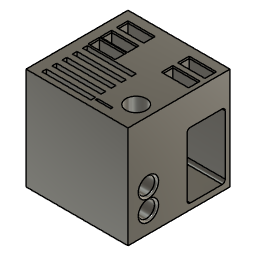
porte_carte_usb v3 (Autodesk Fusion 360 design; units mm, degrees)
Autodesk Fusion 360 part; units mm, degrees
note: some values were not read from the file. Set by a fixed rule: which sketch regions a step uses.
sketch "Esquisse1" plane through (0, 0, 0) normal (0, 0, 1) x (1, 0, 0)
  line L0 (0, 0) -> (50, 0)
  line L1 (50, 0) -> (50, 50)
  line L2 (50, 50) -> (0, 50)
  line L3 (0, 50) -> (0, 0)
  dimension "d1" = 50
  dimension "d2" = 50
  constraint horizontal L0
  constraint vertical L1
  constraint horizontal L2
  constraint vertical L3
  constraint coincident L0.start L3.end
  measures "d1" distance of L0.start L0.end
  measures "d2" distance of L0.start L2.end
extrude "Extrusion1" add sketch "Esquisse1" along normal blind 50
sketch "Esquisse2" plane through (0, 0, 50) normal (0, 0, 1) x (-1, 0, 0)
  line L0 (0, -50) -> (0, 0)
  line L1 (0, 0) -> (-50, 0)
  line L2 (-50, 0) -> (-50, -50)
  line L3 (-50, -50) -> (0, -50)
  line L4 (-5, -45) -> (-17.3, -45)
  line L5 (-17.3, -45) -> (-17.3, -40.4)
  line L6 (-17.3, -40.4) -> (-5, -40.4)
  line L7 (-5, -40.4) -> (-5, -45)
  line L8 (-35, -45) -> (-47.3, -45)
  line L9 (-47.3, -45) -> (-47.3, -40.4)
  line L10 (-47.3, -40.4) -> (-35, -40.4)
  line L11 (-35, -40.4) -> (-35, -45)
  line L12 (-5, -37) -> (-17.3, -37)
  line L13 (-17.3, -37) -> (-17.3, -32.4)
  line L14 (-17.3, -32.4) -> (-5, -32.4)
  line L15 (-5, -32.4) -> (-5, -37)
  line L16 (-35, -37) -> (-47.3, -37)
  line L17 (-47.3, -37) -> (-47.3, -32.4)
  line L18 (-47.3, -32.4) -> (-35, -32.4)
  line L19 (-35, -32.4) -> (-35, -37)
  line L20 (-5, -25) -> (-29, -25)
  line L21 (-29, -25) -> (-29, -22.8)
  line L22 (-29, -22.8) -> (-5, -22.8)
  line L23 (-5, -22.8) -> (-5, -25)
  line L24 (-5, -20) -> (-29, -20)
  line L25 (-29, -20) -> (-29, -17.8)
  line L26 (-29, -17.8) -> (-5, -17.8)
  line L27 (-5, -17.8) -> (-5, -20)
  line L28 (-5, -15) -> (-29, -15)
  line L29 (-29, -15) -> (-29, -12.8)
  line L30 (-29, -12.8) -> (-5, -12.8)
  line L31 (-5, -12.8) -> (-5, -15)
  line L32 (-5, -10) -> (-29, -10)
  line L33 (-29, -10) -> (-29, -7.8)
  line L34 (-29, -7.8) -> (-5, -7.8)
  line L35 (-5, -7.8) -> (-5, -10)
  line L36 (-5, -5) -> (-29, -5)
  line L37 (-29, -5) -> (-29, -2.8)
  line L38 (-29, -2.8) -> (-5, -2.8)
  line L39 (-5, -2.8) -> (-5, -5)
  line L40 (-30, -30) -> (-37, -30)
  line L41 (-37, -30) -> (-37, -29)
  line L42 (-37, -29) -> (-30, -29)
  line L43 (-30, -29) -> (-30, -30)
  line L44 (-41, -30) -> (-47, -30)
  line L45 (-47, -30) -> (-47, -29)
  line L46 (-47, -29) -> (-41, -29)
  line L47 (-41, -29) -> (-41, -30)
  line L48 (-30, -25) -> (-37, -25)
  line L49 (-37, -25) -> (-37, -24)
  line L50 (-37, -24) -> (-30, -24)
  line L51 (-30, -24) -> (-30, -25)
  line L52 (-41, -25) -> (-47, -25)
  line L53 (-47, -25) -> (-47, -24)
  line L54 (-47, -24) -> (-41, -24)
  line L55 (-41, -24) -> (-41, -25)
  line L56 (-30, -20) -> (-37, -20)
  line L57 (-37, -20) -> (-37, -19)
  line L58 (-37, -19) -> (-30, -19)
  line L59 (-30, -19) -> (-30, -20)
  line L60 (-41, -20) -> (-47, -20)
  line L61 (-47, -20) -> (-47, -19)
  line L62 (-47, -19) -> (-41, -19)
  line L63 (-41, -19) -> (-41, -20)
  line L64 (-30, -5) -> (-37.6, -5)
  line L65 (-37.6, -5) -> (-37.6, -4)
  line L66 (-37.6, -4) -> (-30, -4)
  line L67 (-30, -4) -> (-30, -5)
  circle A0 centre (-42, -12) radius 5
  line L68 (-5, -31) -> (-17.3, -31)
  line L69 (-17.3, -31) -> (-17.3, -26.4)
  line L70 (-17.3, -26.4) -> (-5, -26.4)
  line L71 (-5, -26.4) -> (-5, -31)
  circle A1 centre (-33.8, -4.5) radius 0.5
  dimension "d15" = 4.6
  dimension "d16" = 12.3
  dimension "d17" = 12.3
  dimension "d18" = 4.6
  dimension "d19" = 12.3
  dimension "d20" = 4.6
  dimension "d21" = 12.3
  dimension "d22" = 4.6
  dimension "d23" = 24
  dimension "d24" = 2.2
  dimension "d25" = 24
  dimension "d26" = 2.2
  dimension "d27" = 24
  dimension "d28" = 2.2
  dimension "d29" = 24
  dimension "d30" = 2.2
  dimension "d31" = 24
  dimension "d32" = 2.2
  dimension "d33" = 7.6
  dimension "d34" = 1
  dimension "d35" = 12.3
  dimension "d36" = 4.6
  constraint horizontal L4
  constraint vertical L5
  constraint horizontal L6
  constraint vertical L7
  constraint horizontal L8
  constraint vertical L9
  constraint horizontal L10
  constraint vertical L11
  constraint horizontal L12
  constraint vertical L13
  constraint horizontal L14
  constraint vertical L15
  constraint horizontal L16
  constraint vertical L17
  constraint horizontal L18
  constraint vertical L19
  constraint horizontal L20
  constraint vertical L21
  constraint horizontal L22
  constraint vertical L23
  constraint horizontal L24
  constraint vertical L25
  constraint horizontal L26
  constraint vertical L27
  constraint horizontal L28
  constraint vertical L29
  constraint horizontal L30
  constraint vertical L31
  constraint horizontal L32
  constraint vertical L33
  constraint horizontal L34
  constraint vertical L35
  constraint horizontal L36
  constraint vertical L37
  constraint horizontal L38
  constraint vertical L39
  constraint horizontal L40
  constraint vertical L41
  constraint horizontal L42
  constraint vertical L43
  constraint horizontal L44
  constraint vertical L45
  constraint horizontal L46
  constraint vertical L47
  constraint horizontal L48
  constraint vertical L49
  constraint horizontal L50
  constraint vertical L51
  constraint horizontal L52
  constraint vertical L53
  constraint horizontal L54
  constraint vertical L55
  constraint horizontal L56
  constraint vertical L57
  constraint horizontal L58
  constraint vertical L59
  constraint horizontal L60
  constraint vertical L61
  constraint horizontal L62
  constraint vertical L63
  constraint horizontal L64
  constraint vertical L65
  constraint horizontal L66
  constraint vertical L67
  constraint horizontal L68
  constraint vertical L69
  constraint horizontal L70
  constraint vertical L71
  measures "d15" distance of L4.start L6.end
  measures "d16" distance of L4.start L4.end
  measures "d17" distance of L8.start L8.end
  measures "d18" distance of L8.start L10.end
  measures "d19" distance of L12.start L12.end
  measures "d20" distance of L12.start L14.end
  measures "d21" distance of L16.start L16.end
  measures "d22" distance of L16.start L18.end
  measures "d23" distance of L20.start L20.end
  measures "d24" distance of L20.start L22.end
  measures "d25" distance of L24.start L24.end
  measures "d26" distance of L24.start L26.end
  measures "d27" distance of L28.start L28.end
  measures "d28" distance of L28.start L30.end
  measures "d29" distance of L32.start L32.end
  measures "d30" distance of L32.start L34.end
  measures "d31" distance of L36.start L36.end
  measures "d32" distance of L36.start L38.end
  measures "d33" distance of L64.start L64.end
  measures "d34" distance of L64.start L66.end
  measures "d35" distance of L68.start L68.end
  measures "d36" distance of L68.start L70.end
extrude "Extrusion2" cut sketch "Esquisse2" against normal blind 12 contours L4 L5 L6 L7
extrude "Extrusion3" cut sketch "Esquisse2" against normal blind 12 contours L8 L9 L10 L11
extrude "Extrusion4" cut sketch "Esquisse2" against normal blind 12 contours L12 L13 L14 L15 | L16 L17 L18 L19 | L68 L69 L70 L71
extrude "Extrusion5" cut sketch "Esquisse2" against normal blind 23 contours L20 L21 L22 L23 | L24 L25 L26 L27 | L28 L29 L30 L31 | L32 L33 L34 L35 | L36 L37 L38 L39
extrude "Extrusion6" cut sketch "Esquisse2" against normal blind 20 contours A0
extrude "Extrusion7" cut sketch "Esquisse2" against normal blind 22.5 contours A1
extrude "Extrusion8" cut sketch "Esquisse2" against normal blind 13.5 contours L64 L66 L67 A1 | L64 L65 L66 A1
sketch "Esquisse3" plane through (50, 0, 0) normal (1, 0, 0) x (0, 1, 0)
  line L0 (0, 0) -> (50, 0)
  line L1 (50, 0) -> (50, 50)
  line L2 (50, 50) -> (0, 50)
  line L3 (0, 50) -> (0, 0)
  line L4 (29, 35) -> (47.7, 35)
  line L5 (47.7, 35) -> (47.7, 2.9)
  line L6 (47.7, 2.9) -> (29, 2.9)
  line L7 (29, 2.9) -> (29, 35)
  circle A0 centre (10, 10) radius 4
  circle A1 centre (10, 20) radius 4
  dimension "d54" = 18.7
  dimension "d55" = 32.1
  dimension "d64" = 8
  constraint horizontal L4
  constraint vertical L5
  constraint horizontal L6
  constraint vertical L7
  measures "d54" distance of L4.start L4.end
  measures "d55" distance of L4.start L6.end
  measures "d64" diameter of A0
extrude "Extrusion9" cut sketch "Esquisse3" against normal blind 24 contours L4 L5 L6 L7
sketch "Esquisse4" plane through (0, 0, 0) normal (-1, 0, 0) x (0, -1, 0)
  line L0 (-50, 0) -> (0, 0)
  line L1 (0, 0) -> (0, 50)
  line L2 (0, 50) -> (-50, 50)
  line L3 (-50, 50) -> (-50, 0)
  line L4 (-48, 35) -> (-29.3, 35)
  line L5 (-29.3, 35) -> (-29.3, 2.9)
  line L6 (-29.3, 2.9) -> (-48, 2.9)
  line L7 (-48, 2.9) -> (-48, 35)
  dimension "d60" = 18.7
  dimension "d61" = 32.1
  constraint horizontal L4
  constraint vertical L5
  constraint horizontal L6
  constraint vertical L7
  measures "d60" distance of L4.start L4.end
  measures "d61" distance of L4.start L6.end
extrude "Extrusion10" cut sketch "Esquisse4" against normal blind 24 contours L4 L5 L6 L7
extrude "Extrusion11" cut sketch "Esquisse3" against normal blind 50 contours A1
extrude "Extrusion12" cut sketch "Esquisse3" against normal blind 50 contours A0
fillet "Congé1" radius 1.5 4 edges at (38, 29, 35) (38, 47.7, 35) (38, 29, 2.9) (38, 47.7, 2.9)
fillet "Congé2" radius 1.5 4 edges at (12, 48, 35) (12, 29.3, 35) (12, 48, 2.9) (12, 29.3, 2.9)
fillet "Congé3" radius 1 2 edges at (0, 6.2707, 18.5535) (0, 6.2707, 8.5535)
fillet "Congé4" radius 1 2 edges at (50, 6.2707, 21.4465) (50, 6.2707, 11.4465)
chamfer "Chanfrein1" distance 0.5 angle 45 4 edges at (11.15, 31, 50) (5, 28.7, 50) (11.15, 26.4, 50) (17.3, 28.7, 50)
chamfer "Chanfrein2" distance 0.5 angle 45 16 edges at (11.15, 45, 50) (5, 42.7, 50) (11.15, 40.4, 50) (17.3, 42.7, 50) (11.15, 37, 50) (17.3, 34.7, 50) (11.15, 32.4, 50) (5, 34.7, 50) (41.15, 37, 50) (41.15, 32.4, 50) (35, 34.7, 50) (47.3, 34.7, 50) (41.15, 40.4, 50) (47.3, 42.7, 50) (41.15, 45, 50) (35, 42.7, 50)
equation "usb_largeur = 4.6 mm"
equation "usb_longueur = 12.3 mm"
equation "usb_hauteur = 12 mm"
equation "SD_longueur = 24 mm"
equation "SD_largeur = 2.2 mm"
equation "SD_hauteur = 23 mm"
equation "pick_longueur = 7.6 mm"
equation "pick_largeur = 1 mm"
equation "pick_hauteur_1 = 13.5 mm"
equation "pick_hauteur_2 = 9 mm"
equation "d15 = usb_largeur"
equation "d16 = usb_longueur"
equation "d17 = usb_longueur"
equation "d18 = usb_largeur"
equation "d19 = usb_longueur"
equation "d20 = usb_largeur"
equation "d21 = usb_longueur"
equation "d22 = usb_largeur"
equation "d23 = SD_longueur"
equation "d24 = SD_largeur"
equation "d25 = SD_longueur"
equation "d26 = SD_largeur"
equation "d27 = SD_longueur"
equation "d28 = SD_largeur"
equation "d29 = SD_longueur"
equation "d30 = SD_largeur"
equation "d31 = SD_longueur"
equation "d32 = SD_largeur"
equation "d33 = pick_longueur"
equation "d34 = pick_largeur"
equation "d35 = usb_longueur"
equation "d36 = usb_largeur"
equation "d37 = -usb_hauteur"
equation "d39 = -usb_hauteur"
equation "d41 = -usb_hauteur"
equation "d43 = -SD_hauteur"
equation "d47 = -pick_hauteur_1 - pick_hauteur_2"
equation "d49 = -pick_hauteur_1"
equation "batterie_longueur = 32.1 mm"
equation "batterie_largeur = 18.7 mm"
equation "batterie_hauteur = 24 mm"
equation "d54 = batterie_largeur"
equation "d55 = batterie_longueur"
equation "d58 = -batterie_hauteur"
equation "d60 = batterie_largeur"
equation "d61 = batterie_longueur"
equation "d62 = -batterie_hauteur"
